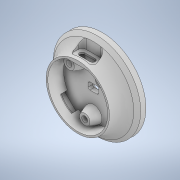
# Autodesk Inventor part: Baseplate
Saved by Autodesk Inventor 2021 (Build 250183000, 183)
## iProperties
Created: 2024-03-24
Part Number: Baseplate
Material: Generic
Document SubType Name: Modeling
Designer: Lukas
Density: 1 g/cm^3
Appearance: Default
Author: Lukas
Autodesk Inventor part; units mm, degrees
ref_plane "XY Plane" through (0, 0, 0) normal (0, 0, 1) x (1, 0, 0)
sketch "Sketch1" plane through (0, 0, 0) normal (0, 0, 1) x (1, 0, 0)
  circle A0 centre (0, 0) radius 25
  circle A1 centre (0, -13) radius 1.65
  circle A2 centre (-9, 10) radius 1.65
  circle A3 centre (9, 10) radius 1.65
  circle A4 centre (-9, 10) radius 3
  circle A5 centre (9, 10) radius 3
  circle A6 centre (0, -13) radius 3
  dimension "d0" = 50
  dimension "d1" = 13
  dimension "d2" = 10
  dimension "d3" = 9
  dimension "d4" = 9
  dimension "d5" = 3.3
  dimension "d6" = 6
  constraints: 7 centre point, 4 coincident, 4 equal radius, 1 horizontal alignment, 1 vertical alignment
  measures "d0" diameter of A0
  measures "d1" distance of point (0, 0) A1.centre
  measures "d2" vertical distance of A3.centre point (0, 0)
  measures "d3" horizontal distance of point (0, 0) A3.centre
  measures "d4" horizontal distance of A2.centre point (0, 0)
  measures "d5" diameter of A2
  measures "d6" diameter of A4
extrude "Extrusion1" add sketch "Sketch1" along normal blind 5 contours A0
extrude "Extrusion2" add sketch "Sketch1" along normal blind 10 contours A4 | A5 | A6
sketch "Sketch2" plane through (0, 0, 0) normal (0, 0, -1) x (-1, 0, 0)
  circle A0 centre (0, -13) radius 1.65 projected
  circle A1 centre (-9, 10) radius 1.65 projected
  circle A2 centre (9, 10) radius 1.65 projected
  circle A3 centre (0, 0) radius 25 projected
  circle A4 centre (-9, 10) radius 3.5
  circle A5 centre (9, 10) radius 3.5
  circle A6 centre (0, -13) radius 3.5
  dimension "d11" = 7
  constraints: 3 centre point, 3 coincident, 2 equal radius
  measures "d11" diameter of A4
extrude "Extrusion3" cut sketch "Sketch2" against normal blind 3 contours A4 | A5 | A6
chamfer "Chamfer1" distance 1.8199 angle 70 3 edges at (-3, -13, 5) (-12, 10, 5) (6, 10, 5) measured on face at (12.0972, -3.5223, 5)
chamfer "Chamfer2" distance 2 angle 45 1 edges at (-25, 0, 5)
sketch "Sketch3" plane through (0, 0, 0) normal (1, 0, 0) x (0, 1, 0)
  line L0 (14.8199, 5) -> (5.1801, 5) projected
  line L1 (-8.1801, 5) -> (-17.8199, 5) projected
  line L2 (14.8199, 5) -> (5.1801, 5) projected
  line L3 (-23, 5) -> (23, 5) projected
  line L4 (25, 0) -> (25, 3) projected
  line L5 (25, 3) -> (-25, 3) projected
  line L6 (-23, 5) -> (23, 5) projected
  line L7 (25, 3) -> (23, 5) projected
  arc A0 (18.1033, 14) -> (23, 5) centre (28.8225, 14) ccw
  line L8 (18.1033, 14) -> (17.1033, 14)
  line L9 (17.1033, 14) -> (17.1033, 5)
  line L10 (0, -3.8) -> (0, 22.8) projected
  point P0 (0, 0)
  dimension "d20" = 9
  dimension "d21" = 18.1033
  dimension "d22" = 1
  constraints: 4 end point, 2 point on circle, 1 centre point, 1 horizontal, 1 line through centre, 1 perpendicular, 1 point on line
  measures "d20" distance of L8.end L9.end
  measures "d21" horizontal distance of point (0, 0) L8.start
  measures "d22" distance of L8.start L8.end
revolve "Revolution1" add sketch "Sketch3" angle 360 about axis through (0, 0, -10) along (0, 0, 1) contours L9 L8 A0 L3
sketch "Sketch5" plane through (0, 0, 14) normal (0, 0, 1) x (1, 0, 0)
  line L0 (4, 17.5) -> (-4, 17.5)
  line L1 (-4, 17.5) -> (-7, 16)
  line L2 (-7, 16) -> (7, 16)
  line L3 (7, 16) -> (4, 17.5)
  point P0 (0, 0)
  point P1 (0, 16)
  point P2 (0, 17.5)
  dimension "d37" = 16
  dimension "d39" = 14
  dimension "d42" = 8
  dimension "d43" = 1.5
  constraints: 8 end point, 2 horizontal, 2 midpoint, 2 vertical alignment
  measures "d37" distance from line of point (0, 0) L2
  measures "d39" distance of L1.end L2.end
  measures "d42" distance of L0.start L0.end
  measures "d43" distance between parallel lines of L2 L0
extrude "Extrusion6" add sketch "Sketch5" against normal up to surface (9 mm away)
ref_plane "Work Plane1" through (0, 25, 0) normal (0, 1, 0) x (-1, 0, 0)
sketch "Sketch4" plane through (0, 25, 0) normal (0, 1, 0) x (-1, 0, 0)
  line L0 (-8.5709, 5) -> (-6.0434, 5) projected
  line L1 (13.8192, 5) -> (8.5709, 5) projected
  line L2 (13.8192, 5) -> (2.8899, 5) projected
  line L3 (-2.8899, 5) -> (2.8899, 5) projected
  line L4 (-2.8899, 5) -> (-13.8192, 5) projected
  line L5 (-8.5709, 5) -> (-13.8192, 5) projected
  line L6 (-3, 8.5) -> (3, 8.5) construction
  line L7 (3.5, 3) -> (-3.5, 3) projected
  line L8 (-4.25, 5) -> (4.25, 5)
  line L9 (4.25, 12) -> (-4.25, 12)
  line L10 (-3, 8.5) -> (3, 8.5) construction
  line L11 (-3, 7) -> (3, 7)
  line L12 (3, 10) -> (-3, 10)
  arc A0 (-3, 10) -> (-3, 7) centre (-3, 8.5) ccw
  arc A1 (3, 7) -> (3, 10) centre (3, 8.5) ccw
  line L13 (-6.0434, 5) -> (6.0434, 5) projected
  line L14 (6.0434, 5) -> (8.5709, 5) projected
  line L15 (-6.5, 9.75) -> (-6.5, 7.25)
  line L16 (6.5, 7.25) -> (6.5, 9.75)
  arc A2 (-4.25, 12) -> (-6.5, 9.75) centre (-4.25, 9.75) ccw
  arc A3 (-6.5, 7.25) -> (-4.25, 5) centre (-4.25, 7.25) ccw
  arc A4 (4.25, 5) -> (6.5, 7.25) centre (4.25, 7.25) ccw
  arc A5 (6.5, 9.75) -> (4.25, 12) centre (4.25, 9.75) ccw
  point P0 (0, 0)
  point P1 (0, 5)
  point P2 (0, 8.5)
  point P3 (0, 5)
  point P4 (0, 8.5)
  point P5 (6.5, 8.5)
  point P6 (0, 12)
  dimension "d30" = 7
  dimension "d32" = 3.5
  dimension "d33" = 3
  dimension "d34" = 9
  dimension "d52" = 13
  dimension "d53" = 2.25
  constraints: 20 end point, 12 point on circle, 12 tangent, 6 centre point, 5 midpoint, 3 equal radius, 3 parallel, 2 horizontal, 2 vertical, 2 vertical alignment, 1 coincident, 1 horizontal alignment, 1 point on line
  measures "d30" distance between parallel lines of L8 L9
  measures "d32" distance from line of L0 point (0, 8.5)
  measures "d33" distance between parallel lines of L11 L12
  measures "d52" distance between parallel lines of L16 L15
  measures "d53" radius of A2
extrude "Extrusion4" cut sketch "Sketch4" against normal blind 10 contours A0 L12 A1 L11
extrude "Extrusion5" cut sketch "Sketch4" against normal blind 8
sketch "Sketch6" plane through (0, 0, 5) normal (0, 0, 1) x (1, 0, 0)
  line L0 (-2, 2) -> (2, 2)
  line L1 (3, 1) -> (3, -1)
  line L2 (2, -2) -> (-2, -2)
  line L3 (-3, -1) -> (-3, 1)
  arc A0 (-2, 2) -> (-3, 1) centre (-2, 1) ccw
  arc A1 (3, 1) -> (2, 2) centre (2, 1) ccw
  arc A2 (2, -2) -> (3, -1) centre (2, -1) ccw
  arc A3 (-3, -1) -> (-2, -2) centre (-2, -1) ccw
  point P0 (0, 0)
  point P1 (0, 2)
  point P2 (-3, 0)
  dimension "d44" = 1
  dimension "d45" = 4
  dimension "d46" = 6
  constraints: 8 end point, 8 point on circle, 8 tangent, 4 centre point, 3 equal radius, 2 midpoint, 2 parallel, 1 horizontal, 1 horizontal alignment, 1 perpendicular, 1 vertical alignment
  measures "d44" radius of A0
  measures "d45" distance between parallel lines of L2 L0
  measures "d46" distance between parallel lines of L3 L1
extrude "Extrusion7" cut sketch "Sketch6" against normal through all
chamfer "Chamfer3" distance 2.5 angle 45 8 edges at (0, 2, 0) (-2.7071, 1.7071, 0) (-3, 0, 0) (-2.7071, -1.7071, 0) (0, -2, 0) (2.7071, -1.7071, 0) (3, 0, 0) (2.7071, 1.7071, 0)
ref_plane "Work Plane2" through (0, 0, 0) normal (0.7071068, 0.7071068, 0) x (0, 0, 1)
sketch "Sketch7" plane through (0, 0, 0) normal (0.7071068, 0.7071068, 0) x (0, 0, 1)
  line L0 (5, -4.5) -> (7, -4.5)
  line L1 (7, -4.5) -> (7, 4.5)
  line L2 (7, 4.5) -> (5, 4.5)
  line L3 (5, 4.5) -> (5, -4.5)
  line L4 (5, -16.8974) -> (5, 9.8765) projected
  point P0 (0, 0)
  point P1 (5, 0)
  dimension "d54" = 9
  dimension "d55" = 2
  constraints: 8 end point, 2 parallel, 1 horizontal, 1 horizontal alignment, 1 midpoint, 1 perpendicular, 1 point on line
  measures "d54" distance of L0.end L1.end
  measures "d55" distance of L0.start L0.end
extrude "Extrusion8" cut sketch "Sketch7" against normal blind 18.75
chamfer "Chamfer4" distance 2.17 angle 45 1 edges at (-12.0938, -12.0938, 7)
equation "\"d4\" = d3"
body "Solid1"
